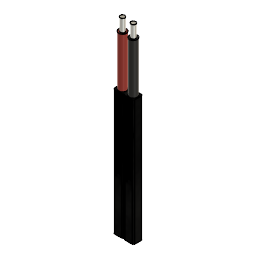
Wire End (FA1) (Autodesk Fusion 360 design; units mm, degrees)
Autodesk Fusion 360 part; units mm, degrees
sketch "Sketch1" plane through (0, 0, 0) normal (0, 0, 1) x (1, 0, 0)
  line L0 (1.625, -0.55) -> (1.625, 0.55)
  arc A0 (-1.625, -0.55) -> (-1.425, -0.75) centre (-1.425, -0.55) ccw
  line L1 (-1.625, 0.55) -> (-1.625, -0.55)
  arc A1 (-1.425, 0.75) -> (-1.625, 0.55) centre (-1.425, 0.55) ccw
  arc A2 (1.425, -0.75) -> (1.625, -0.55) centre (1.425, -0.55) ccw
  line L2 (1.625, -0.75) -> (-1.625, 0.75) construction
  line L3 (-1.625, -0.75) -> (1.625, 0.75) construction
  arc A3 (1.625, 0.55) -> (1.425, 0.75) centre (1.425, 0.55) ccw
  arc A4 (-0.1231, 0.6643) -> (0.1231, 0.6643) centre (0, 0.75) ccw
  line L4 (1.425, 0.75) -> (0.2872, 0.75)
  line L5 (-0.2872, 0.75) -> (-1.425, 0.75)
  arc A5 (0.1129, -0.6643) -> (-0.1333, -0.6643) centre (-0.0102, -0.75) ccw
  line L6 (-1.425, -0.75) -> (-0.2975, -0.75)
  line L7 (0.277, -0.75) -> (1.425, -0.75)
  arc A6 (-0.1231, 0.6643) -> (-0.2872, 0.75) centre (-0.2872, 0.55) ccw
  arc A7 (0.2872, 0.75) -> (0.1231, 0.6643) centre (0.2872, 0.55) ccw
  arc A8 (0.1129, -0.6643) -> (0.277, -0.75) centre (0.277, -0.55) ccw
  arc A9 (-0.2975, -0.75) -> (-0.1333, -0.6643) centre (-0.2975, -0.55) ccw
  dimension "d15" = 3.25
  dimension "d16" = 1.5
  dimension "d17" = 0.2
  dimension "d18" = 0.2
  dimension "d19" = 0.3
  dimension "d20" = 0.3
  dimension "d21" = 0.2
  constraint perpendicular L0 L6
  constraint parallel L4 L6
  constraint parallel L0 L1
  constraint coincident origin L3
  constraint coincident origin L2
  constraint coincident L2.start L6
  constraint coincident L2.start L0
  constraint tangent A2 L6
  constraint tangent L0 A2
  constraint coincident L3.start L1
  constraint coincident L3.start L6
  constraint tangent A0 L1
  constraint tangent A0 L6
  constraint equal A0 A2
  constraint coincident L2.end L1
  constraint coincident L2.end L4
  constraint tangent L1 A1
  constraint tangent A1 L4
  constraint equal A1 A2
  constraint coincident L3.end L4
  constraint coincident L3.end L0
  constraint tangent A3 L4
  constraint tangent L0 A3
  constraint collinear L4 L5
  constraint coincident A4.centre L4
  constraint collinear L6 L7
  constraint coincident A5.centre L6
  constraint tangent A4 A6
  constraint tangent L5 A6
  constraint tangent A4 A7
  constraint tangent L4 A7
  constraint equal A6 A7
  constraint tangent A5 A8
  constraint tangent L7 A8
  constraint equal A6 A8
  constraint tangent A5 A9
  constraint tangent L6 A9
  constraint equal A6 A9
  measures "d15" distance of L3.end L2.end
  measures "d16" distance of L3.end L2.start
  measures "d17" radius of A2
  measures "d18" radius of A3
  measures "d19" diameter of A4
  measures "d20" diameter of A5
  measures "d21" radius of A6
extrude "Extrude1" add sketch "Sketch1" along normal blind 20 makes body 1
sketch "Sketch2" plane through (0, 0, 20) normal (0, 0, 1) x (-1, 0, 0)
  line L0 (0, 0) -> (-0.866, 0) construction
  line L1 (0, 0) -> (0.866, 0) construction
  circle A0 centre (-0.866, 0) radius 0.625
  circle A1 centre (0.866, 0) radius 0.625
  line L2 (0.2872, -0.75) -> (1.425, -0.75)
  arc A2 (1.425, -0.75) -> (1.625, -0.55) centre (1.425, -0.55) ccw
  line L3 (1.625, -0.55) -> (1.625, 0.55)
  arc A3 (1.625, 0.55) -> (1.425, 0.75) centre (1.425, 0.55) ccw
  line L4 (1.425, 0.75) -> (0.2975, 0.75)
  arc A4 (-1.425, 0.75) -> (-1.625, 0.55) centre (-1.425, 0.55) ccw
  line L5 (-1.625, 0.55) -> (-1.625, -0.55)
  arc A5 (-1.625, -0.55) -> (-1.425, -0.75) centre (-1.425, -0.55) ccw
  arc A6 (0.1231, -0.6643) -> (0.2872, -0.75) centre (0.2872, -0.55) ccw
  arc A7 (0.2975, 0.75) -> (0.1333, 0.6643) centre (0.2975, 0.55) ccw
  arc A8 (-0.1129, 0.6643) -> (0.1333, 0.6643) centre (0.0102, 0.75) ccw
  arc A9 (-0.1129, 0.6643) -> (-0.277, 0.75) centre (-0.277, 0.55) ccw
  line L6 (-0.277, 0.75) -> (-1.425, 0.75)
  line L7 (-1.425, -0.75) -> (-0.2872, -0.75)
  arc A10 (-0.2872, -0.75) -> (-0.1231, -0.6643) centre (-0.2872, -0.55) ccw
  arc A11 (0.1231, -0.6643) -> (-0.1231, -0.6643) centre (0, -0.75) ccw
  dimension "d5" = 0.866
  dimension "d6" = 0.866
  dimension "d7" = 1.25
  dimension "d8" = 1.25
  constraint coincident L0.start L1.start
  constraint horizontal L0
  constraint parallel L0 L1
  constraint coincident L0.end A0.centre
  constraint coincident L1.end A1.centre
  measures "d5" distance of L0.start L0.end
  measures "d6" distance of L0.start L1.end
  measures "d7" diameter of A0
  measures "d8" diameter of A1
extrude "Extrude2" add sketch "Sketch2" along normal blind 8 separate body contours A0 | A1 makes body 2 at (-1.4879, 0.0622, 22.6667) makes body 3 at (0.2441, 0.0622, 22.6667)
sketch "Sketch3" plane through (0, 0, 28) normal (0, 0, 1) x (-1, 0, 0)
  circle A0 centre (0.866, 0) radius 0.625
  circle A1 centre (0.866, 0) radius 0.375
  dimension "d11" = 0.75
  constraint concentric A0 A1
  measures "d11" diameter of A1
sketch "Sketch4" plane through (0, 0, 28) normal (0, 0, 1) x (-1, 0, 0)
  circle A0 centre (-0.866, 0) radius 0.625
  circle A1 centre (-0.866, 0) radius 0.375
  dimension "d12" = 0.75
  constraint concentric A0 A1
  measures "d12" diameter of A1
extrude "Extrude3" add sketch "Sketch4" sketch "Sketch3" along normal blind 2 separate body contours A1 of sketch 2 contours A1 makes body 4 at (0.4929, 0.0373, 28.6667) makes body 5 at (-1.2392, 0.0373, 28.6667)
equation "d5 = 1.73205081 mm / 2"
equation "d6 = 1.73205081 mm / 2"
